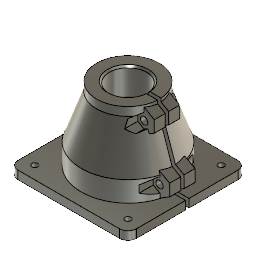
pipe-bearing-holder (Autodesk Fusion 360 design; units mm, degrees)
Autodesk Fusion 360 part; units mm, degrees
sketch "Sketch1" plane through (0, 0, 0) normal (0, 0, 1) x (1, 0, 0)
  line L0 (0, 0) -> (70, 0)
  line L1 (70, 0) -> (70, 70)
  line L2 (70, 70) -> (0, 70)
  line L3 (0, 70) -> (0, 0)
  circle A0 centre (7.5, 62.5) radius 1.75
  circle A1 centre (62.5, 62.5) radius 1.75
  circle A2 centre (7.5, 7.5) radius 1.75
  circle A3 centre (62.5, 7.5) radius 1.75
  dimension "d1" = 70
  dimension "d2" = 70
  dimension "d3" = 3.5
  dimension "d4" = 7.5
  dimension "d5" = 7.5
  dimension "d8" = 55
  dimension "d9" = -55
  measures "d1" distance of L0.start L2.end
  measures "d2" distance of L0.start L0.end
  measures "d3" diameter of A0
  measures "d4" distance of L3 A0.centre
  measures "d5" distance of L2 A0.centre
extrude "Extrude1" add sketch "Sketch1" along normal blind 5
sketch "Sketch3" plane through (0, 0, 5) normal (0, 0, 1) x (-1, 0, 0)
  circle A0 centre (-62.5, -62.5) radius 1.75
  circle A1 centre (-7.5, -62.5) radius 1.75
  circle A2 centre (-7.5, -7.5) radius 1.75
  circle A3 centre (-62.5, -7.5) radius 1.75
  line L0 (0, -70) -> (0, 0)
  line L1 (0, 0) -> (-70, 0)
  line L2 (-70, 0) -> (-70, -70)
  line L3 (-70, -70) -> (0, -70)
  circle A4 centre (-35, -35) radius 20.15
  dimension "d15" = 40.3
  measures "d15" diameter of A4
extrude "Extrude2" cut sketch "Sketch3" against normal blind 10 contours A4
sketch "Sketch4" plane through (0, 0, 5) normal (0, 0, 1) x (-1, 0, 0)
  circle A0 centre (-35, -35) radius 20.15
  circle A1 centre (-62.5, -62.5) radius 1.75
  circle A2 centre (-7.5, -62.5) radius 1.75
  circle A3 centre (-7.5, -7.5) radius 1.75
  circle A4 centre (-62.5, -7.5) radius 1.75
  line L0 (0, -70) -> (0, 0)
  line L1 (0, 0) -> (-70, 0)
  line L2 (-70, 0) -> (-70, -70)
  line L3 (-70, -70) -> (0, -70)
  circle A5 centre (-35, -35) radius 27.5
  dimension "d18" = 55
  measures "d18" diameter of A5
extrude "Extrude3" add sketch "Sketch4" along normal blind 12 contours A5
ref_plane "WorkPlane2" through (35, 35, 2.5) normal (0, -1, 0) x (1, 0, 0)
sketch "Sketch7" plane through (35, 35, 2.5) normal (0, -1, 0) x (1, 0, 0)
  line L0 (27.5, 14.5) -> (-27.5, 14.5)
  line L1 (27.5, 14.5) -> (20.15, 14.5)
  line L2 (20.15, -2.5) -> (-20.15, -2.5)
  line L3 (0, 0) -> (0, 65)
  line L4 (11, 29.5) -> (11, 45.5)
  line L5 (11, 45.5) -> (18.5, 45.5)
  line L6 (18.5, 45.5) -> (18.5, 40.5)
  line L7 (20.15, 14.5) -> (11, 29.5)
  line L8 (27.5, 14.5) -> (18.5, 40.5)
  point P0 (27.5, 14.5)
  point P1 (20.15, 14.5)
  dimension "d27" = 11
  dimension "d28" = 7.5
  dimension "d29" = 16
  dimension "d30" = 15
  dimension "d31" = 5
  measures "d27" distance of L3 L4
  measures "d28" distance of L4 L6
  measures "d29" distance of L4.start L4.end
  measures "d30" distance of P1 L4.start
  measures "d31" distance of L5.end L6.end
revolve "Revolve1" add sketch "Sketch7" angle 360 about axis through (35, 35, 2.5) along (0, 0, 1)
sketch "Sketch11" plane through (35, 35, 2.5) normal (0, -1, 0) x (1, 0, 0)
  line L0 (35, -2.5) -> (-35, -2.5)
  line L1 (20.15, 14.5) -> (20.15, -2.5)
  line L2 (20.1145, 9.5) -> (32.1145, 9.5)
  line L3 (32.0551, 13.065) -> (25.9974, 16.4272)
  line L4 (25.9974, 16.4272) -> (20.0568, 12.8622)
  line L5 (20.0568, 12.8622) -> (20.174, 5.935)
  line L6 (20.174, 5.935) -> (26.2317, 2.5728)
  line L7 (26.2317, 2.5728) -> (32.1722, 6.1378)
  line L8 (32.1722, 6.1378) -> (32.0551, 13.065)
  point P0 (20.15, 14.5)
  point P1 (20.15, -2.5)
  point P2 (26.1145, 9.5)
  dimension "d41" = 12
  dimension "d49" = 6
  dimension "d51" = 6
  measures "d41" distance of P1 L2
  measures "d49" distance of P2 L3
  measures "d51" distance of L2.start P2
extrude "Extrude5" add sketch "Sketch11" along normal mid plane 15
sketch "Sketch12" plane through (0, 27.5, 0) normal (0, -1, 0) x (1, 0, 0)
  line L0 (61.4575, 17) -> (61.4575, 5.2083)
  line L1 (61.4575, 5.2083) -> (67.1722, 8.6378)
  line L2 (67.1722, 8.6378) -> (67.0551, 15.565)
  line L3 (67.0551, 15.565) -> (60.9974, 18.9272)
  line L4 (67.1137, 12.1014) -> (61.1149, 11.9768)
  circle A0 centre (61.1149, 11.9768) radius 2.15
  line L5 (60.9974, 18.9272) -> (61.2317, 5.0728)
  line L6 (60.9974, 18.9272) -> (60.805, 18.8118)
  spline S0 degree 2 poles (61.4575, 17) (61.1275, 17.9172) (60.805, 18.8118) knots 0 0 0 0.192415 0.192415 0.192415 weights 1 1.000077 1.000009
  point P0 (60.9974, 18.9272)
  point P1 (61.2317, 5.0728)
  dimension "d44" = 4.3
  measures "d44" diameter of A0
extrude "Extrude6" cut sketch "Sketch12" along normal mid plane 60 contours L0 L4 A0 | L0 L4 A0 L5 | L0 L4 A0 | L0 L4 A0 L5 | A0 L5
sketch "Sketch13" plane through (0, 27.5, 0) normal (0, -1, 0) x (1, 0, 0)
  arc A0 (61.4575, 9.8543) -> (61.4575, 14.0993) centre (61.1149, 11.9768) ccw
  line L0 (61.4575, 9.8543) -> (61.4575, 5.2083)
  line L1 (61.4575, 5.2083) -> (67.1722, 8.6378)
  line L2 (67.1722, 8.6378) -> (67.0551, 15.565)
  line L3 (67.0551, 15.565) -> (60.9974, 18.9272)
  line L4 (61.4575, 17) -> (61.4575, 14.0993)
  line L5 (64.8125, 14.1172) -> (61.1101, 16.2492)
  line L6 (61.1101, 16.2492) -> (57.4125, 14.1088)
  line L7 (57.4125, 14.1088) -> (57.4173, 9.8364)
  line L8 (57.4173, 9.8364) -> (61.1197, 7.7044)
  line L9 (61.1197, 7.7044) -> (64.8173, 9.8448)
  line L10 (64.8173, 9.8448) -> (64.8125, 14.1172)
  line L11 (60.9974, 18.9272) -> (60.805, 18.8118)
  spline S0 degree 2 poles (61.4575, 17) (61.1275, 17.9172) (60.805, 18.8118) knots 0 0 0 0.192415 0.192415 0.192415 weights 1 1.000077 1.000009
  point P0 (61.1149, 11.9768)
  dimension "d65" = 3.7
  measures "d65" distance of P0 L10
extrude "Extrude7" cut sketch "Sketch13" along normal blind 10 contours A0 L0 L4 L5 L6 L7 L8 L9
sketch "Sketch14" plane through (0, 42.5, 0) normal (0, 1, 0) x (-1, 0, 0)
  arc A0 (-61.4575, 14.0993) -> (-61.4575, 9.8543) centre (-61.1149, 11.9768) ccw
  line L0 (-61.4575, 14.0993) -> (-61.4575, 17)
  line L1 (-60.9974, 18.9272) -> (-67.0551, 15.565)
  line L2 (-67.0551, 15.565) -> (-67.1722, 8.6378)
  line L3 (-67.1722, 8.6378) -> (-61.4575, 5.2083)
  line L4 (-61.4575, 5.2083) -> (-61.4575, 9.8543)
  circle A1 centre (-61.1149, 11.9768) radius 4
  spline S0 degree 2 poles (-60.805, 18.8118) (-61.1275, 17.9172) (-61.4575, 17) knots 0.012424 0.012424 0.012424 0.204839 0.204839 0.204839 weights 1.000009 1.000077 1
  line L5 (-60.805, 18.8118) -> (-60.9974, 18.9272)
  dimension "d52" = 8
  measures "d52" diameter of A1
extrude "Extrude8" cut sketch "Sketch14" along normal blind 19.5 contours A0 L0 L4 A1 picked at (-60.01, 11.9768)
sketch "Sketch15" plane through (35, 35, 2.5) normal (0, -1, 0) x (1, 0, 0)
  line L0 (-18.5, 40.5) -> (18.5, 40.5)
  line L1 (11, 45.5) -> (11, 29.5)
  line L2 (11, 29.5) -> (11, 37.5)
  line L3 (11, 37.5) -> (24, 37.5)
  line L4 (23, 40.9641) -> (17, 44.4282)
  line L5 (17, 44.4282) -> (11, 40.9641)
  line L6 (11, 40.9641) -> (11, 34.0359)
  line L7 (11, 34.0359) -> (17, 30.5718)
  line L8 (17, 30.5718) -> (23, 34.0359)
  line L9 (23, 34.0359) -> (23, 40.9641)
  point P0 (11, 45.5)
  point P1 (11, 29.5)
  point P2 (17, 37.5)
  dimension "d55" = 6
  dimension "d72" = 6
  measures "d55" distance of L2.end P2
  measures "d72" distance of P2 L4
extrude "Extrude9" add sketch "Sketch15" along normal mid plane 15
sketch "Sketch16" plane through (0, 27.5, 0) normal (0, -1, 0) x (1, 0, 0)
  spline S0 degree 2 poles (54.9799, 34.7922) (53.3363, 39.2374) (51.9115, 43) knots 0.169143 0.169143 0.169143 1.05964 1.05964 1.05964 weights 1.001132 1.003546 1
  line L0 (54.9799, 34.7922) -> (58, 36.5359)
  line L1 (58, 36.5359) -> (58, 43.4641)
  line L2 (58, 43.4641) -> (52, 46.9282)
  line L3 (52, 46.9282) -> (51.9115, 46.8771)
  line L4 (51.9115, 46.8771) -> (51.9115, 43)
  line L5 (52, 46.9282) -> (52, 38.8216)
  line L6 (58, 40) -> (52, 40)
  circle A0 centre (52, 40) radius 2.15
  dimension "d58" = 4.3
  measures "d58" diameter of A0
extrude "Extrude10" cut sketch "Sketch16" along normal mid plane 60 contours S0 L5 L6 A0 | S0 L6 A0 | S0 L5 L6 A0 | S0 L6 A0
sketch "Sketch17" plane through (0, 27.5, 0) normal (0, -1, 0) x (1, 0, 0)
  arc A0 (53.585, 38.5474) -> (52.2379, 42.1368) centre (52, 40) ccw
  spline S0 degree 2 poles (54.9799, 34.7922) (54.2605, 36.7377) (53.585, 38.5474) knots 0.169143 0.169143 0.169143 0.558347 0.558347 0.558347 weights 1.001132 1.002187 1.002104
  line L0 (54.9799, 34.7922) -> (58, 36.5359)
  line L1 (58, 36.5359) -> (58, 43.4641)
  line L2 (58, 43.4641) -> (52, 46.9282)
  line L3 (52, 46.9282) -> (51.9115, 46.8771)
  line L4 (51.9115, 46.8771) -> (51.9115, 43)
  spline S1 degree 2 poles (52.2379, 42.1368) (52.0734, 42.5725) (51.9115, 43) knots 0.958785 0.958785 0.958785 1.05964 1.05964 1.05964 weights 1.000727 1.000402 1
  line L5 (55.7, 42.1362) -> (52, 44.2724)
  line L6 (52, 44.2724) -> (48.3, 42.1362)
  line L7 (48.3, 42.1362) -> (48.3, 37.8638)
  line L8 (48.3, 37.8638) -> (52, 35.7276)
  line L9 (52, 35.7276) -> (55.7, 37.8638)
  line L10 (55.7, 37.8638) -> (55.7, 42.1362)
  point P0 (52, 40)
  dimension "d74" = 7.4
  measures "d74" distance of L5 L8
extrude "Extrude11" cut sketch "Sketch17" along normal blind 18 contours A0 S0 L4 S1 L6 L7 L8 L9 | A0 S0 L4 S1 L5 L6 L9 L10
sketch "Sketch18" plane through (0, 42.5, 0) normal (0, 1, 0) x (-1, 0, 0)
  arc A0 (-52.2379, 42.1368) -> (-53.585, 38.5474) centre (-52, 40) ccw
  spline S0 degree 2 poles (-51.9115, 43) (-52.0734, 42.5725) (-52.2379, 42.1368) knots 0 0 0 0.100855 0.100855 0.100855 weights 1 1.000402 1.000727
  line L0 (-51.9115, 43) -> (-51.9115, 46.8771)
  line L1 (-51.9115, 46.8771) -> (-52, 46.9282)
  line L2 (-52, 46.9282) -> (-58, 43.4641)
  line L3 (-58, 43.4641) -> (-58, 36.5359)
  line L4 (-58, 36.5359) -> (-54.9799, 34.7922)
  spline S1 degree 2 poles (-53.585, 38.5474) (-54.2605, 36.7377) (-54.9799, 34.7922) knots 0.501293 0.501293 0.501293 0.890497 0.890497 0.890497 weights 1.002104 1.002187 1.001132
  circle A1 centre (-52, 40) radius 4
  dimension "d73" = 8
  measures "d73" diameter of A1
extrude "Extrude12" cut sketch "Sketch18" along normal blind 14 contours A0 S0 L0 S1 A1 | A0 S0 L0 S1 A1
sketch "Sketch19" plane through (70, 0, 0) normal (1, 0, 0) x (0, 1, 0)
  line L0 (0, 0) -> (70, 0)
  line L1 (70, 0) -> (70, 5)
  line L2 (70, 5) -> (0, 5)
  line L3 (0, 5) -> (0, 0)
  line L4 (34, 0) -> (36, 0)
  line L5 (36, 0) -> (36, 59.3349)
  line L6 (36, 59.3349) -> (34, 59.3349)
  line L7 (34, 59.3349) -> (34, 0)
  dimension "d66" = 2
  dimension "d67" = 34
  measures "d66" distance of L5.end L6.end
  measures "d67" distance of L3 L7
extrude "Extrude13" cut sketch "Sketch19" against normal blind 30 contours L0 L2 L4 L5 L7 | L2 L5 L6 L7
fillet "Fillet3" radius 5 4 edges at (70, 70, 2.5) (0, 70, 2.5) (0, 0, 2.5) (70, 0, 2.5)
chamfer "Chamfer1" distance 1 angle 45 2 edges at (24, 35, 48) (14.85, 35, 0)
